Autodesk Fusion 360 part; units mm, degrees
(part 16 of 25)
  arc A4441 (68.687, 0.8538) -> (68.3831, 0.9459) centre (68.535, 0.8998) ccw
  line L1561 (83.8624, 50.0146) -> (84.0359, 50.3392)
  arc A4442 (68.3648, 3.5705) -> (68.6582, 3.692) centre (68.5115, 3.6312) ccw
  line L1562 (68.4422, 3.7777) -> (68.3972, 3.8451)
  arc A4443 (68.6582, 0.7615) -> (68.3648, 0.883) centre (68.5115, 0.8222) ccw
  arc A4444 (83.2647, 49.041) -> (83.0633, 49.2864) centre (83.164, 49.1637) ccw
  arc A4445 (33.749, 4.337) -> (33.749, 4.0195) centre (33.749, 4.1783) ccw
  line L1563 (67.8546, 4.1703) -> (67.7739, 4.1783)
  arc A4446 (33.3467, 3.8529) -> (33.1222, 4.0774) centre (33.2345, 3.9652) ccw
  line L1564 (33.1257, 3.8451) -> (33.0806, 3.7777)
  arc A4447 (67.839, 4.0124) -> (67.8702, 4.3283) centre (67.8546, 4.1704) ccw
  arc A4448 (32.8647, 3.692) -> (33.158, 3.5705) centre (33.0114, 3.6312) ccw
  line L1565 (33.0424, 3.7062) -> (33.0113, 3.6312)
  line L1566 (33.749, 4.1783) -> (33.6683, 4.1703)
  arc A4449 (32.9024, 3.781) -> (33.1824, 3.6313) centre (33.0424, 3.7062) ccw
  arc A4450 (32.8359, 3.5997) -> (33.1397, 3.5075) centre (32.9878, 3.5536) ccw
  line L1567 (68.0118, 4.131) -> (67.9342, 4.1545)
  arc A4451 (33.6527, 4.3283) -> (33.6838, 4.0124) centre (33.6683, 4.1704) ccw
  line L1568 (68.2257, 4.0166) -> (68.1582, 4.0617)
  arc A4452 (67.7894, 4.3363) -> (67.7583, 4.0203) centre (67.7739, 4.1783) ccw
  line L1569 (68.1582, 4.0617) -> (68.0867, 4.0999)
  arc A4453 (67.9802, 4.3064) -> (67.8881, 4.0026) centre (67.9341, 4.1545) ccw
  line L1570 (33.4362, 4.0999) -> (33.3646, 4.0617)
  line L1571 (33.0806, 3.7777) -> (33.0424, 3.7062)
  arc A4454 (33.2577, 3.7569) -> (32.9937, 3.9333) centre (33.1257, 3.8451) ccw
  arc A4455 (33.3754, 4.2466) -> (33.4969, 3.9533) centre (33.4361, 4.0999) ccw
  line L1572 (33.3646, 4.0617) -> (33.2972, 4.0166)
  arc A4456 (32.9486, 3.8659) -> (33.2126, 3.6895) centre (33.0806, 3.7777) ccw
  arc A4457 (68.2335, 3.7956) -> (68.458, 4.0201) centre (68.3458, 3.9079) ccw
  arc A4458 (33.3979, 3.8939) -> (33.1965, 4.1394) centre (33.2972, 4.0167) ccw
  arc A4459 (83.3016, 49.5247) -> (83.547, 49.3233) centre (83.4243, 49.424) ccw
  line L1573 (33.1771, 3.9078) -> (33.1257, 3.8451)
  arc A4460 (33.2998, 3.8071) -> (33.0544, 4.0085) centre (33.1771, 3.9078) ccw
  arc A4461 (33.6348, 4.0026) -> (33.5426, 4.3064) centre (33.5887, 4.1545) ccw
  arc A4462 (33.2206, 3.7029) -> (32.9406, 3.8525) centre (33.0806, 3.7777) ccw
  line L1574 (67.9342, 4.1545) -> (67.8546, 4.1703)
  arc A4463 (33.7645, 4.0203) -> (33.7334, 4.3363) centre (33.749, 4.1783) ccw
  arc A4464 (68.1375, 3.8846) -> (68.3139, 4.1486) centre (68.2257, 4.0166) ccw
  arc A4465 (67.7739, 4.0195) -> (67.7739, 4.337) centre (67.7739, 4.1783) ccw
  arc A4466 (68.0834, 3.9217) -> (68.2331, 4.2017) centre (68.1583, 4.0617) ccw
  arc A4467 (33.5718, 3.9843) -> (33.4503, 4.2776) centre (33.5111, 4.131) ccw
  arc A4468 (33.189, 3.6454) -> (32.8957, 3.7669) centre (33.0423, 3.7062) ccw
  arc A4469 (33.2898, 4.2017) -> (33.4395, 3.9217) centre (33.3646, 4.0617) ccw
  arc A4470 (33.511, 3.9599) -> (33.3613, 4.2399) centre (33.4362, 4.0999) ccw
  arc A4471 (33.6992, 4.0146) -> (33.6373, 4.326) centre (33.6683, 4.1703) ccw
  line L1575 (33.5887, 4.1545) -> (33.5111, 4.131)
  arc A4472 (33.209, 4.1486) -> (33.3854, 3.8846) centre (33.2972, 4.0166) ccw
  arc A4473 (68.0725, 4.2776) -> (67.951, 3.9843) centre (68.0118, 4.1309) ccw
  line L1576 (84.1767, 50.6793) -> (84.2253, 50.8394)
  arc A4474 (33.1633, 3.5852) -> (32.8594, 3.6773) centre (33.0114, 3.6312) ccw
  line L1577 (68.2884, 3.9652) -> (68.2257, 4.0166)
  arc A4475 (68.1615, 4.2399) -> (68.0119, 3.9599) centre (68.0867, 4.0999) ccw
  line L1578 (67.7739, 4.1783) -> (33.749, 4.1783)
  arc A4476 (67.9657, 3.9791) -> (68.0579, 4.2829) centre (68.0118, 4.131) ccw
  line L1579 (33.0113, 3.6312) -> (32.9878, 3.5536)
  arc A4477 (67.9032, 3.9988) -> (67.9651, 4.3102) centre (67.9342, 4.1545) ccw
  arc A4478 (33.465, 4.2829) -> (33.5572, 3.9791) centre (33.5111, 4.131) ccw
  arc A4479 (33.1338, 4.0879) -> (33.3352, 3.8425) centre (33.2345, 3.9652) ccw
  arc A4480 (33.4528, 3.9297) -> (33.2764, 4.1937) centre (33.3646, 4.0617) ccw
  arc A4481 (68.1877, 3.8425) -> (68.3891, 4.0879) centre (68.2884, 3.9652) ccw
  line L1580 (33.6683, 4.1703) -> (33.5887, 4.1545)
  line L1581 (33.2972, 4.0166) -> (33.2345, 3.9652)
  arc A4482 (68.3264, 4.1394) -> (68.125, 3.8939) centre (68.2257, 4.0166) ccw
  arc A4483 (33.0649, 4.0201) -> (33.2894, 3.7956) centre (33.1772, 3.9079) ccw
  line L1582 (33.2345, 3.9652) -> (33.1771, 3.9078)
  arc A4484 (68.026, 3.9533) -> (68.1475, 4.2466) centre (68.0867, 4.1) ccw
  arc A4485 (33.5577, 4.3102) -> (33.6197, 3.9988) centre (33.5887, 4.1545) ccw
  arc A4486 (1.1732, 49.6203) -> (1.4371, 49.7967) centre (1.3051, 49.7085) ccw
  line L1583 (0.7863, 50.6793) -> (0.9271, 50.3392)
  arc A4487 (0.9266, 50.7635) -> (0.6228, 50.6713) centre (0.7747, 50.7174) ccw
  arc A4488 (33.122, 1.0757) -> (32.806, 1.0446) centre (32.964, 1.0601) ccw
  line L1584 (32.964, 1.0601) -> (32.972, 0.9794)
  arc A4489 (0.9329, 50.7401) -> (0.6396, 50.6186) centre (0.7863, 50.6793) ccw
  arc A4490 (32.814, 0.9638) -> (33.13, 0.995) centre (32.972, 0.9794) ccw
  arc A4491 (32.806, 3.4089) -> (33.122, 3.3778) centre (32.964, 3.3933) ccw
  line L1585 (3.0543, 48.4113) -> (3.4066, 48.3044)
  line L1586 (1.1006, 50.0146) -> (1.3052, 49.7085)
  arc A4492 (1.6867, 49.0514) -> (1.9112, 49.2759) centre (1.799, 49.1637) ccw
  arc A4493 (32.8844, 0.7139) -> (33.1777, 0.8355) centre (33.0311, 0.7747) ccw
  arc A4494 (3.3605, 48.1525) -> (3.4527, 48.4563) centre (3.4066, 48.3044) ccw
  arc A4495 (33.13, 3.4585) -> (32.814, 3.4896) centre (32.972, 3.4741) ccw
  line L1587 (2.0835, 48.9302) -> (2.3896, 48.7256)
  line L1588 (1.5387, 49.424) -> (1.799, 49.1637)
  arc A4496 (1.8997, 49.2864) -> (1.6983, 49.041) centre (1.799, 49.1637) ccw
  arc A4497 (3.4375, 48.4601) -> (3.3756, 48.1487) centre (3.4065, 48.3044) ccw
  line L1589 (0.7747, 0.7747) -> (0.7747, 50.7174)
  arc A4498 (32.8321, 0.8689) -> (33.1435, 0.9308) centre (32.9878, 0.8998) ccw
  arc A4499 (33.031, 0.6159) -> (33.031, 0.9334) centre (33.031, 0.7747) ccw
  arc A4500 (1.2326, 50.1028) -> (0.9686, 49.9264) centre (1.1006, 50.0146) ccw
  arc A4501 (32.8594, 0.7761) -> (33.1633, 0.8683) centre (33.0114, 0.8222) ccw
  arc A4502 (68.2464, 4.1937) -> (68.07, 3.9297) centre (68.1582, 4.0617) ccw
  arc A4503 (33.003, 3.9458) -> (33.2484, 3.7444) centre (33.1257, 3.8451) ccw
  arc A4504 (33.158, 0.883) -> (32.8647, 0.7615) centre (33.0114, 0.8222) ccw
  arc A4505 (33.1397, 0.9459) -> (32.8359, 0.8538) centre (32.9878, 0.8999) ccw
  line L1590 (3.4066, 48.3044) -> (3.7676, 48.2326)
  arc A4506 (1.416, 49.3233) -> (1.6614, 49.5247) centre (1.5387, 49.424) ccw
  arc A4507 (1.9828, 48.8074) -> (2.1842, 49.0529) centre (2.0835, 48.9301) ccw
  arc A4508 (0.7805, 50.2785) -> (1.0738, 50.4) centre (0.9272, 50.3392) ccw
  line L1591 (2.3896, 48.7256) -> (2.7142, 48.5521)
  line L1592 (32.9878, 0.8998) -> (33.0113, 0.8222)
  arc A4509 (1.6509, 49.5362) -> (1.4264, 49.3117) centre (1.5387, 49.424) ccw
  arc A4510 (2.6394, 48.4121) -> (2.7891, 48.6921) centre (2.7143, 48.5521) ccw
  line L1593 (33.5111, 4.131) -> (33.4362, 4.0999)
  arc A4511 (3.7366, 48.0769) -> (3.7986, 48.3883) centre (3.7676, 48.2326) ccw
  arc A4512 (2.4644, 48.8656) -> (2.3148, 48.5856) centre (2.3896, 48.7256) ccw
  arc A4513 (33.1435, 3.5227) -> (32.8321, 3.5846) centre (32.9878, 3.5537) ccw
  line L1594 (1.799, 49.1637) -> (2.0835, 48.9302)
  arc A4514 (33.1277, 1.0104) -> (32.8163, 0.9484) centre (32.972, 0.9794) ccw
  line L1595 (2.7142, 48.5521) -> (3.0543, 48.4113)
  line L1596 (68.0867, 4.0999) -> (68.0118, 4.131)
  arc A4515 (1.4279, 49.8092) -> (1.1824, 49.6078) centre (1.3051, 49.7085) ccw
  arc A4516 (2.1717, 49.0621) -> (1.9953, 48.7982) centre (2.0835, 48.9302) ccw
  line L1597 (33.0113, 0.8222) -> (33.031, 0.7747)
  arc A4517 (32.8163, 3.505) -> (33.1277, 3.4431) centre (32.972, 3.474) ccw
  arc A4518 (32.8053, 1.0601) -> (33.1228, 1.0601) centre (32.9641, 1.0601) ccw
  line L1598 (33.031, 0.7747) -> (0.7747, 0.7747)
  arc A4519 (3.1004, 48.5632) -> (3.0082, 48.2593) centre (3.0543, 48.4113) ccw
  arc A4520 (2.3014, 48.5936) -> (2.4778, 48.8576) centre (2.3896, 48.7256) ccw
  arc A4521 (0.9334, 50.7174) -> (0.6159, 50.7174) centre (0.7747, 50.7174) ccw
  arc A4522 (67.8856, 4.326) -> (67.8236, 4.0146) centre (67.8546, 4.1703) ccw
  line L1599 (0.9271, 50.3392) -> (1.1006, 50.0146)
  arc A4523 (0.6343, 50.6332) -> (0.9382, 50.7254) centre (0.7863, 50.6793) ccw
  line L1600 (1.3052, 49.7085) -> (1.5387, 49.424)
  arc A4524 (2.9936, 48.2646) -> (3.1151, 48.5579) centre (3.0543, 48.4112) ccw
  arc A4525 (0.9606, 49.9398) -> (1.2406, 50.0894) centre (1.1006, 50.0146) ccw
  line L1601 (3.7676, 48.2326) -> (4.0005, 48.2096)
  arc A4526 (0.6159, 0.7747) -> (0.9334, 0.7747) centre (0.7747, 0.7747) ccw
  arc A4527 (33.1228, 3.3934) -> (32.8053, 3.3934) centre (32.9641, 3.3934) ccw
  arc A4528 (8.1085, 50.9855) -> (7.8047, 51.0777) centre (7.9566, 51.0316) ccw
  arc A4529 (8.0514, 52.1017) -> (8.0514, 52.4192) centre (8.0514, 52.2604) ccw
  arc A4530 (4.6199, 48.3676) -> (4.6511, 48.0517) centre (4.6355, 48.2097) ccw
  arc A4531 (3.9849, 48.0517) -> (4.0161, 48.3676) centre (4.0005, 48.2097) ccw
  arc A4532 (4.4768, 51.6255) -> (4.7943, 51.6255) centre (4.6356, 51.6255) ccw
  line L1602 (0.7747, 50.7174) -> (0.7863, 50.6793)
  arc A4533 (7.2096, 49.3117) -> (6.9851, 49.5362) centre (7.0974, 49.424) ccw
  arc A4534 (4.1593, 51.6255) -> (3.8418, 51.6255) centre (4.0005, 51.6255) ccw
  arc A4535 (4.4767, 48.2096) -> (4.7942, 48.2096) centre (4.6355, 48.2096) ccw
  arc A4536 (5.6278, 48.2593) -> (5.5356, 48.5632) centre (5.5817, 48.4113) ccw
  line L1603 (4.6355, 48.2096) -> (4.8684, 48.2326)
  line L1604 (4.0005, 48.2096) -> (4.0005, 51.6255)
  arc A4537 (1.0671, 50.4141) -> (0.7871, 50.2644) centre (0.9271, 50.3392) ccw
  arc A4538 (4.8839, 48.0746) -> (4.8528, 48.3906) centre (4.8683, 48.2326) ccw
  arc A4539 (7.3953, 50.0894) -> (7.6754, 49.9398) centre (7.5353, 50.0146) ccw
  arc A4540 (4.6355, 51.7843) -> (4.6355, 51.4668) centre (4.6355, 51.6256) ccw
  line L1605 (4.6355, 51.6255) -> (4.6355, 52.2605)
  line L1606 (7.9566, 51.0316) -> (8.0284, 51.3926)
  arc A4541 (7.9964, 50.6186) -> (7.7031, 50.7401) centre (7.8498, 50.6793) ccw
  arc A4542 (4.0005, 51.7842) -> (4.0005, 51.4667) centre (4.0005, 51.6255) ccw
  arc A4543 (3.7832, 48.3906) -> (3.752, 48.0746) centre (3.7676, 48.2326) ccw
  line L1607 (5.5817, 48.4113) -> (5.9218, 48.5521)
  arc A4544 (4.7943, 52.2605) -> (4.4768, 52.2605) centre (4.6356, 52.2605) ccw
  line L1608 (4.6355, 52.2605) -> (8.0514, 52.2605)
  arc A4545 (4.6355, 51.4667) -> (4.6355, 51.7842) centre (4.6355, 51.6255) ccw
  line L1609 (4.0005, 51.6255) -> (4.6355, 51.6255)
  line L1610 (32.972, 0.9794) -> (32.9878, 0.8998)
  arc A4546 (6.3212, 48.5856) -> (6.1716, 48.8656) centre (6.2464, 48.7256) ccw
  line L1611 (6.2464, 48.7256) -> (6.5525, 48.9302)
  arc A4547 (6.9746, 49.5247) -> (7.22, 49.3233) centre (7.0973, 49.424) ccw
  arc A4548 (5.8469, 48.6921) -> (5.9966, 48.4121) centre (5.9218, 48.5521) ccw
  arc A4549 (8.2093, 51.6099) -> (7.8934, 51.6411) centre (8.0513, 51.6255) ccw
  arc A4550 (6.4518, 49.0529) -> (6.6532, 48.8074) centre (6.5525, 48.9301) ccw
  line L1612 (32.964, 3.3934) -> (32.964, 1.0601)
  arc A4551 (7.8704, 51.4082) -> (8.1864, 51.377) centre (8.0284, 51.3926) ccw
  arc A4552 (3.8418, 48.2096) -> (4.1593, 48.2096) centre (4.0005, 48.2096) ccw
  line L1613 (7.8497, 50.6793) -> (7.9566, 51.0316)
  line L1614 (7.3308, 49.7085) -> (7.5354, 50.0146)
  arc A4553 (5.5209, 48.5579) -> (5.6424, 48.2646) centre (5.5816, 48.4112) ccw
  arc A4554 (8.1841, 51.3616) -> (7.8727, 51.4236) centre (8.0284, 51.3926) ccw
  arc A4555 (4.8374, 48.3883) -> (4.8994, 48.0769) centre (4.8684, 48.2326) ccw
  arc A4556 (7.8009, 51.0625) -> (8.1123, 51.0006) centre (7.9566, 51.0316) ccw
  line L1615 (5.2294, 48.3044) -> (5.5817, 48.4113)
  arc A4557 (7.8489, 50.2644) -> (7.5689, 50.4141) centre (7.7089, 50.3392) ccw
  arc A4558 (0.7747, 0.9334) -> (0.7747, 0.6159) centre (0.7747, 0.7747) ccw
  arc A4559 (7.6978, 50.7254) -> (8.0017, 50.6332) centre (7.8498, 50.6793) ccw
  line L1616 (32.9878, 3.5536) -> (32.972, 3.4741)
  line L1617 (7.5354, 50.0146) -> (7.7089, 50.3392)
  arc A4560 (8.0514, 51.4668) -> (8.0514, 51.7843) centre (8.0514, 51.6256) ccw
  line L1618 (32.972, 3.4741) -> (32.964, 3.3934)
  line L1619 (5.9218, 48.5521) -> (6.2464, 48.7256)
  line L1620 (8.0284, 51.3926) -> (8.0514, 51.6255)
  line L1621 (8.0514, 51.6255) -> (4.6355, 51.6255)
  arc A4561 (6.7248, 49.2759) -> (6.9493, 49.0514) centre (6.8371, 49.1637) ccw
  line L1622 (4.8684, 48.2326) -> (5.2294, 48.3044)
  arc A4562 (5.1833, 48.4563) -> (5.2755, 48.1525) centre (5.2294, 48.3044) ccw
  arc A4563 (2.775, 48.6988) -> (2.6535, 48.4055) centre (2.7143, 48.5522) ccw
  arc A4564 (5.2604, 48.1487) -> (5.1985, 48.4601) centre (5.2294, 48.3044) ccw
  line L1623 (6.837, 49.1637) -> (7.0973, 49.424)
  arc A4565 (4.7942, 51.6255) -> (4.4767, 51.6255) centre (4.6355, 51.6255) ccw
  line L1624 (7.0973, 49.424) -> (7.3308, 49.7085)
  arc A4566 (7.6673, 49.9264) -> (7.4034, 50.1028) centre (7.5353, 50.0146) ccw
  arc A4567 (71.3694, 40.4649) -> (71.3694, 40.7824) centre (71.3694, 40.6237) ccw
  line L1625 (70.4098, 40.4328) -> (70.3249, 40.3479)
  arc A4568 (7.4536, 49.6078) -> (7.2081, 49.8092) centre (7.3309, 49.7085) ccw
  arc A4569 (5.4611, 55.6772) -> (5.3689, 55.3734) centre (5.415, 55.5253) ccw
  arc A4570 (6.4643, 54.8238) -> (6.6407, 55.0878) centre (6.5525, 54.9558) ccw
  arc A4571 (72.227, 39.5586) -> (72.5204, 39.6801) centre (72.3737, 39.6194) ccw
  arc A4572 (70.3491, 40.5795) -> (70.4706, 40.2862) centre (70.4099, 40.4329) ccw
  arc A4573 (7.6754, 53.9462) -> (7.3953, 53.7966) centre (7.5353, 53.8714) ccw
  arc A4574 (6.6532, 55.0786) -> (6.4518, 54.8331) centre (6.5525, 54.9558) ccw
  line L1626 (6.837, 54.7223) -> (6.5525, 54.9558)
  line L1627 (7.7089, 53.5468) -> (7.5354, 53.8714)
  line L1628 (4.6355, 51.6255) -> (4.6355, 48.2096)
  arc A4575 (6.3346, 55.2923) -> (6.1582, 55.0284) centre (6.2464, 55.1604) ccw
  line L1629 (6.2464, 55.1604) -> (5.9218, 55.3339)
  arc A4576 (7.8555, 53.6075) -> (7.5622, 53.486) centre (7.7088, 53.5468) ccw
  arc A4577 (7.22, 54.5627) -> (6.9746, 54.3613) centre (7.0973, 54.462) ccw
  line L1630 (5.9218, 55.3339) -> (5.5817, 55.4747)
  arc A4578 (5.6424, 55.6214) -> (5.5209, 55.3281) centre (5.5816, 55.4748) ccw
  arc A4579 (6.6407, 48.7982) -> (6.4643, 49.0621) centre (6.5525, 48.9301) ccw
  arc A4580 (7.4628, 54.2657) -> (7.1988, 54.0893) centre (7.3308, 54.1775) ccw
  arc A4581 (70.8706, 40.7824) -> (70.8706, 40.4649) centre (70.8706, 40.6237) ccw
  arc A4582 (70.2126, 40.4602) -> (70.4372, 40.2356) centre (70.3249, 40.3479) ccw
  arc A4583 (8.0017, 53.2528) -> (7.6978, 53.1606) centre (7.8497, 53.2067) ccw
  line L1631 (6.5525, 54.9558) -> (6.2464, 55.1604)
  line L1632 (7.5354, 53.8714) -> (7.3308, 54.1775)
  arc A4584 (7.8934, 52.2449) -> (8.2093, 52.2761) centre (8.0514, 52.2605) ccw
  arc A4585 (6.1582, 48.8576) -> (6.3346, 48.5936) centre (6.2464, 48.7256) ccw
  arc A4586 (72.0706, 39.9679) -> (72.2951, 40.1924) centre (72.1829, 40.0802) ccw
  arc A4587 (8.1123, 52.8854) -> (7.8009, 52.8235) centre (7.9566, 52.8545) ccw
  line L1633 (70.8706, 40.6237) -> (70.4098, 40.4328)
  arc A4588 (6.7363, 54.5996) -> (6.9377, 54.845) centre (6.837, 54.7223) ccw
  line L1634 (8.0284, 52.4934) -> (7.9566, 52.8544)
  arc A4589 (6.9377, 49.041) -> (6.7363, 49.2864) centre (6.837, 49.1637) ccw
  arc A4590 (70.5221, 40.3206) -> (70.2976, 40.5451) centre (70.4099, 40.4329) ccw
  arc A4591 (8.1864, 52.5089) -> (7.8704, 52.4778) centre (8.0284, 52.4934) ccw
  arc A4592 (7.5689, 53.4719) -> (7.8489, 53.6216) centre (7.7089, 53.5468) ccw
  arc A4593 (7.7031, 53.1459) -> (7.9964, 53.2674) centre (7.8498, 53.2067) ccw
  line L1635 (5.5817, 55.4747) -> (5.415, 55.5253)
  arc A4594 (6.9493, 54.8346) -> (6.7248, 54.6101) centre (6.8371, 54.7224) ccw
  arc A4595 (72.2149, 39.1206) -> (72.5324, 39.1206) centre (72.3736, 39.1206) ccw
  arc A4596 (5.9825, 48.4055) -> (5.861, 48.6988) centre (5.9218, 48.5522) ccw
  arc A4597 (7.8727, 52.4624) -> (8.1841, 52.5244) centre (8.0284, 52.4934) ccw
  arc A4598 (5.9966, 55.4739) -> (5.8469, 55.1939) centre (5.9217, 55.3339) ccw
  line L1636 (8.0514, 52.2605) -> (8.0284, 52.4934)
  arc A4599 (5.861, 55.1872) -> (5.9825, 55.4805) centre (5.9218, 55.3338) ccw
  arc A4600 (70.9314, 40.477) -> (70.8099, 40.7704) centre (70.8706, 40.6237) ccw
  line L1637 (5.415, 55.5253) -> (79.548, 55.5253)
  arc A4601 (5.5356, 55.3228) -> (5.6278, 55.6267) centre (5.5817, 55.4748) ccw
  arc A4602 (7.5622, 50.4) -> (7.8555, 50.2785) centre (7.7088, 50.3392) ccw
  line L1638 (71.3694, 40.6237) -> (70.8706, 40.6237)
  line L1639 (7.7089, 50.3392) -> (7.8497, 50.6793)
  line L1640 (7.3308, 54.1775) -> (7.0973, 54.462)
  line L1641 (72.3737, 39.1206) -> (72.3737, 39.6194)
  arc A4603 (72.5324, 39.6194) -> (72.2149, 39.6194) centre (72.3736, 39.6194) ccw
  line L1642 (6.5525, 48.9302) -> (6.837, 49.1637)
  arc A4604 (4.6355, 52.4192) -> (4.6355, 52.1017) centre (4.6355, 52.2604) ccw
  line L1643 (7.0973, 54.462) -> (6.837, 54.7223)
  arc A4605 (79.548, 55.3666) -> (79.548, 55.684) centre (79.548, 55.5253) ccw
  arc A4606 (7.1988, 49.7967) -> (7.4628, 49.6203) centre (7.3308, 49.7085) ccw
  line L1644 (72.3737, 39.6194) -> (72.1828, 40.0802)
  arc A4607 (7.8047, 52.8083) -> (8.1085, 52.9005) centre (7.9566, 52.8544) ccw
  arc A4608 (72.3295, 40.1409) -> (72.0362, 40.0194) centre (72.1829, 40.0802) ccw
  line L1645 (52.2859, 37.4845) -> (52.2859, 38.2029)
  arc A4609 (52.4446, 38.2029) -> (52.1271, 38.2029) centre (52.2858, 38.2029) ccw
  line L1646 (52.2859, 38.2029) -> (52.4751, 38.3921)
  arc A4610 (51.9362, 40.2012) -> (51.8147, 40.4946) centre (51.8755, 40.3479) ccw
  arc A4611 (50.0723, 36.5018) -> (50.2968, 36.7264) centre (50.1845, 36.6141) ccw
  arc A4612 (6.1716, 55.0203) -> (6.3212, 55.3004) centre (6.2464, 55.1604) ccw
  arc A4613 (71.7694, 40.2862) -> (71.8909, 40.5795) centre (71.8302, 40.4329) ccw
  arc A4614 (52.1271, 37.4845) -> (52.4446, 37.4845) centre (52.2858, 37.4845) ccw
  line L1647 (50.9029, 39.5859) -> (50.1845, 39.5859)
  line L1648 (52.4751, 38.3921) -> (70.3249, 38.3921)
  arc A4615 (70.3249, 38.2334) -> (70.3249, 38.5508) centre (70.3249, 38.3921) ccw
  arc A4616 (52.4751, 38.5508) -> (52.4751, 38.2334) centre (52.4751, 38.3921) ccw
  line L1649 (72.1828, 38.6598) -> (72.3737, 39.1206)
  line L1650 (71.3694, 38.1163) -> (71.8302, 38.3072)
  arc A4617 (50.1845, 36.7728) -> (50.1845, 36.4554) centre (50.1845, 36.6141) ccw
  arc A4618 (52.5873, 38.2798) -> (52.3628, 38.5044) centre (52.4751, 38.3921) ccw
  arc A4619 (52.3982, 37.3723) -> (52.1736, 37.5968) centre (52.2859, 37.4846) ccw
  arc A4620 (51.6283, 40.0868) -> (51.4038, 40.3113) centre (51.516, 40.199) ccw
  arc A4621 (52.1736, 38.3152) -> (52.3982, 38.0907) centre (52.2859, 38.203) ccw
  arc A4622 (70.4372, 38.5044) -> (70.2126, 38.2798) centre (70.3249, 38.3921) ccw
  arc A4623 (51.4155, 36.4554) -> (51.4155, 36.7728) centre (51.4155, 36.6141) ccw
  arc A4624 (49.4264, 37.5968) -> (49.2018, 37.3723) centre (49.3141, 37.4846) ccw
  line L1651 (70.4098, 38.3072) -> (70.8706, 38.1163)
  line L1652 (50.1845, 36.6141) -> (51.4155, 36.6141)
  arc A4625 (70.4706, 38.4538) -> (70.3491, 38.1605) centre (70.4099, 38.3072) ccw
  arc A4626 (70.8099, 37.9696) -> (70.9314, 38.263) centre (70.8706, 38.1163) ccw
  arc A4627 (50.7907, 39.6982) -> (51.0152, 39.4736) centre (50.903, 39.5859) ccw
  line L1653 (53.34, 17.78) -> (53.34, 19.2405)
  line L1654 (53.34, 19.2405) -> (53.34, 17.78)
  line L1655 (71.8302, 40.4328) -> (71.3694, 40.6237)
  line L1656 (51.5161, 40.199) -> (51.241, 39.9239)
  arc A4628 (71.4301, 40.7704) -> (71.3086, 40.477) centre (71.3693, 40.6237) ccw
  line L1657 (7.9566, 52.8544) -> (7.8497, 53.2067)
  arc A4629 (70.8706, 38.2751) -> (70.8706, 37.9576) centre (70.8706, 38.1164) ccw
  arc A4630 (72.2951, 38.5476) -> (72.0706, 38.7721) centre (72.1829, 38.6599) ccw
  line L1658 (51.8755, 40.3479) -> (51.5161, 40.199)
  line L1659 (70.8706, 38.1163) -> (71.3694, 38.1163)
  line L1660 (7.8497, 53.2067) -> (7.7089, 53.5468)
  arc A4631 (71.7179, 38.4194) -> (71.9424, 38.1949) centre (71.8302, 38.3072) ccw
  arc A4632 (49.2018, 38.8277) -> (49.4264, 38.6032) centre (49.3141, 38.7155) ccw
  arc A4633 (53.4988, 19.2405) -> (53.1813, 19.2405) centre (53.3401, 19.2405) ccw
  arc A4634 (70.3249, 40.1891) -> (70.3249, 40.5066) centre (70.3249, 40.3479) ccw
  arc A4635 (51.1287, 40.0362) -> (51.3532, 39.8117) centre (51.241, 39.924) ccw
  arc A4636 (71.3086, 38.263) -> (71.4301, 37.9696) centre (71.3693, 38.1163) ccw
  arc A4637 (50.9029, 39.4271) -> (50.9029, 39.7446) centre (50.9029, 39.5859) ccw
  arc A4638 (7.4034, 53.7832) -> (7.6673, 53.9596) centre (7.5353, 53.8714) ccw
  arc A4639 (51.3532, 39.8117) -> (51.1287, 40.0362) centre (51.241, 39.924) ccw
  arc A4640 (70.2976, 38.1949) -> (70.5221, 38.4194) centre (70.4099, 38.3072) ccw
  arc A4641 (7.2081, 54.0768) -> (7.4536, 54.2782) centre (7.3308, 54.1775) ccw
  arc A4642 (71.9424, 40.5451) -> (71.7179, 40.3206) centre (71.8302, 40.4328) ccw
  line L1661 (72.1828, 40.0802) -> (71.8302, 40.4328)
  arc A4643 (5.415, 55.684) -> (5.415, 55.3666) centre (5.415, 55.5253) ccw
  arc A4644 (51.8755, 40.5066) -> (51.8755, 40.1891) centre (51.8755, 40.3479) ccw
  arc A4645 (71.3694, 37.9576) -> (71.3694, 38.2751) centre (71.3694, 38.1164) ccw
  arc A4646 (6.9851, 54.3498) -> (7.2096, 54.5743) centre (7.0974, 54.4621) ccw
  line L1662 (49.3141, 37.4845) -> (50.1845, 36.6141)
  arc A4647 (50.2968, 39.4736) -> (50.0723, 39.6982) centre (50.1846, 39.5859) ccw
  arc A4648 (50.1845, 39.7446) -> (50.1845, 39.4271) centre (50.1845, 39.5859) ccw
  arc A4649 (51.3032, 36.7264) -> (51.5277, 36.5018) centre (51.4154, 36.6141) ccw
  arc A4650 (53.4987, 19.2405) -> (53.1812, 19.2405) centre (53.34, 19.2405) ccw
  line L1663 (70.3249, 40.3479) -> (51.8755, 40.3479)
  line L1664 (51.241, 39.9239) -> (50.9029, 39.5859)
  line L1665 (50.1845, 39.5859) -> (49.3141, 38.7155)
  arc A4651 (28.1833, 34.8511) -> (28.4079, 35.0756) centre (28.2956, 34.9634) ccw
  arc A4652 (53.945, 19.0817) -> (53.945, 19.3992) centre (53.945, 19.2405) ccw
  arc A4653 (53.34, 17.9388) -> (53.34, 17.6213) centre (53.34, 17.78) ccw
  line L1666 (49.3141, 38.7155) -> (49.3141, 37.4845)
  arc A4654 (16.5671, 14.6245) -> (16.8846, 14.6245) centre (16.7259, 14.6245) ccw
  line L1667 (25.0444, 37.4267) -> (25.6921, 36.779)
  line L1668 (27.3433, 39.7256) -> (25.9967, 39.7256)
  line L1669 (25.0444, 34.9633) -> (25.0444, 33.6167)
  arc A4655 (51.7104, 19.0868) -> (51.8319, 19.3801) centre (51.7712, 19.2334) ccw
  arc A4656 (27.4891, 35.611) -> (27.8066, 35.611) centre (27.6479, 35.611) ccw
  arc A4657 (28.4543, 34.9633) -> (28.1368, 34.9633) centre (28.2956, 34.9633) ccw
  line L1670 (70.3249, 38.3921) -> (70.4098, 38.3072)
  arc A4658 (25.5798, 36.6667) -> (25.8044, 36.8912) centre (25.6921, 36.779) ccw
  line L1671 (52.2496, 18.7551) -> (51.7712, 19.2335)
  line L1672 (50.459, 19.4945) -> (49.8288, 19.2335)
  line L1673 (52.735, 19.2405) -> (52.2496, 18.7551)
  arc A4659 (46.4368, 21.5237) -> (46.6613, 21.7482) centre (46.549, 21.636) ccw
  arc A4660 (27.3433, 39.5668) -> (27.3433, 39.8843) centre (27.3433, 39.7256) ccw
  arc A4661 (72.0362, 38.7206) -> (72.3295, 38.5991) centre (72.1829, 38.6599) ccw
  arc A4662 (46.2739, 22.0698) -> (46.2739, 21.7523) centre (46.2739, 21.9111) ccw
  arc A4663 (25.5333, 35.611) -> (25.8509, 35.611) centre (25.6921, 35.611) ccw
  line L1674 (25.6921, 36.779) -> (25.6921, 35.611)
  line L1675 (28.2956, 38.7733) -> (27.3433, 39.7256)
  arc A4664 (25.8044, 35.4988) -> (25.5798, 35.7233) centre (25.6921, 35.6111) ccw
  arc A4665 (28.1368, 37.4267) -> (28.4543, 37.4267) centre (28.2956, 37.4267) ccw
  arc A4666 (24.8856, 33.6167) -> (25.2032, 33.6167) centre (25.0444, 33.6167) ccw
  arc A4667 (72.5204, 39.0599) -> (72.227, 39.1814) centre (72.3737, 39.1206) ccw
  arc A4668 (50.459, 19.6532) -> (50.459, 19.3357) centre (50.459, 19.4945) ccw
  arc A4669 (51.141, 19.3357) -> (51.141, 19.6532) centre (51.141, 19.4945) ccw
  arc A4670 (51.8834, 19.3457) -> (51.6589, 19.1212) centre (51.7712, 19.2335) ccw
  line L1676 (27.3433, 32.6644) -> (28.2956, 33.6167)
  arc A4671 (27.2311, 32.7767) -> (27.4556, 32.5521) centre (27.3434, 32.6644) ccw
  arc A4672 (28.1368, 33.6167) -> (28.4543, 33.6167) centre (28.2956, 33.6167) ccw
  arc A4673 (52.1373, 18.6428) -> (52.3619, 18.8673) centre (52.2496, 18.755) ccw
  arc A4674 (49.7681, 19.3801) -> (49.8896, 19.0868) centre (49.8289, 19.2335) ccw
  arc A4675 (50.5197, 19.3478) -> (50.3982, 19.6412) centre (50.459, 19.4945) ccw
  line L1677 (51.7712, 19.2335) -> (51.141, 19.4945)
  arc A4676 (52.735, 19.3992) -> (52.735, 19.0817) centre (52.735, 19.2405) ccw
  arc A4677 (51.2018, 19.6412) -> (51.0803, 19.3478) centre (51.1411, 19.4945) ccw
  line L1678 (71.8302, 38.3072) -> (72.1828, 38.6598)
  arc A4678 (49.1554, 37.4845) -> (49.4729, 37.4845) centre (49.3142, 37.4845) ccw
  arc A4679 (27.8066, 36.779) -> (27.4891, 36.779) centre (27.6479, 36.779) ccw
  line L1679 (27.6479, 36.779) -> (28.2956, 37.4267)
  line L1680 (51.141, 19.4945) -> (50.459, 19.4945)
  arc A4680 (52.8473, 19.1282) -> (52.6228, 19.3528) centre (52.7351, 19.2405) ccw
  arc A4681 (53.1813, 17.78) -> (53.4988, 17.78) centre (53.3401, 17.78) ccw
  line L1681 (51.4155, 36.6141) -> (52.2859, 37.4845)
  arc A4682 (53.34, 19.0817) -> (53.34, 19.3992) centre (53.34, 19.2405) ccw
  arc A4683 (71.8909, 38.1605) -> (71.7694, 38.4538) centre (71.8302, 38.3072) ccw
  arc A4684 (52.1373, 18.8673) -> (52.3619, 18.6428) centre (52.2496, 18.7551) ccw
  line L1682 (53.34, 19.2405) -> (52.735, 19.2405)
  arc A4685 (53.1812, 17.78) -> (53.4987, 17.78) centre (53.34, 17.78) ccw
  arc A4686 (27.4556, 39.8379) -> (27.2311, 39.6133) centre (27.3434, 39.7256) ccw
  arc A4687 (12.7062, 34.7907) -> (12.4129, 34.9122) centre (12.5596, 34.8514) ccw
  arc A4688 (49.4729, 38.7155) -> (49.1554, 38.7155) centre (49.3142, 38.7155) ccw
  arc A4689 (14.6245, 16.8846) -> (14.6245, 16.5671) centre (14.6245, 16.7259) ccw
  arc A4690 (51.4553, 40.3457) -> (51.5768, 40.0524) centre (51.516, 40.1991) ccw
  arc A4691 (53.34, 17.6213) -> (53.34, 17.9388) centre (53.34, 17.78) ccw
  line L1683 (25.9967, 32.6644) -> (27.3433, 32.6644)
  line L1684 (15.8555, 16.7259) -> (14.6245, 16.7259)
  arc A4692 (14.7368, 16.6136) -> (14.5123, 16.8382) centre (14.6245, 16.7259) ccw
  arc A4693 (15.9677, 16.8382) -> (15.7432, 16.6136) centre (15.8555, 16.7259) ccw
  arc A4694 (16.8846, 15.8555) -> (16.5671, 15.8555) centre (16.7259, 15.8555) ccw
  line L1685 (7.62, 21.59) -> (7.62, 23.4315)
  line L1686 (14.6245, 16.7259) -> (13.7541, 15.8555)
  arc A4695 (7.7787, 21.59) -> (7.4612, 21.59) centre (7.62, 21.59) ccw
  line L1687 (13.7541, 15.8555) -> (13.7541, 14.6245)
  line L1688 (5.7785, 22.3528) -> (5.7785, 21.59)
  arc A4696 (13.6418, 15.9677) -> (13.8664, 15.7432) centre (13.7541, 15.8554) ccw
  arc A4697 (28.1833, 38.6611) -> (28.4079, 38.8856) centre (28.2956, 38.7734) ccw
  arc A4698 (15.8555, 13.5954) -> (15.8555, 13.9129) centre (15.8555, 13.7542) ccw
  arc A4699 (9.3027, 20.8272) -> (9.6202, 20.8272) centre (9.4615, 20.8272) ccw
  line L1689 (6.8572, 23.4315) -> (5.7785, 22.3528)
  line L1690 (25.9967, 39.7256) -> (25.0444, 38.7733)
  arc A4700 (25.9967, 39.8843) -> (25.9967, 39.5668) centre (25.9967, 39.7256) ccw
  line L1691 (25.0444, 38.7733) -> (25.0444, 37.4267)
  arc A4701 (25.1567, 33.7289) -> (24.9321, 33.5044) centre (25.0444, 33.6167) ccw
  arc A4702 (7.62, 21.4312) -> (7.62, 21.7487) centre (7.62, 21.59) ccw
  arc A4703 (25.8509, 36.779) -> (25.5333, 36.779) centre (25.6921, 36.779) ccw
  arc A4704 (25.8844, 32.5521) -> (26.1089, 32.7767) centre (25.9966, 32.6644) ccw
  arc A4705 (28.4079, 37.3144) -> (28.1833, 37.5389) centre (28.2956, 37.4267) ccw
  arc A4706 (24.9321, 38.8856) -> (25.1567, 38.6611) centre (25.0444, 38.7734) ccw
  arc A4707 (28.4543, 38.7733) -> (28.1368, 38.7733) centre (28.2956, 38.7733) ccw
  line L1692 (25.6921, 35.611) -> (25.0444, 34.9633)
  arc A4708 (26.1089, 39.6133) -> (25.8844, 39.8379) centre (25.9966, 39.7256) ccw
  arc A4709 (27.3433, 32.5057) -> (27.3433, 32.8231) centre (27.3433, 32.6644) ccw
  arc A4710 (25.2032, 34.9633) -> (24.8856, 34.9633) centre (25.0444, 34.9633) ccw
  line L1693 (27.6479, 35.611) -> (27.6479, 36.779)
  arc A4711 (16.6136, 15.7432) -> (16.8382, 15.9677) centre (16.7259, 15.8554) ccw
  arc A4712 (25.9967, 32.8231) -> (25.9967, 32.5057) centre (25.9967, 32.6644) ccw
  line L1694 (28.2956, 33.6167) -> (28.2956, 34.9633)
  line L1695 (16.7259, 14.6245) -> (16.7259, 15.8555)
  arc A4713 (27.7602, 35.7233) -> (27.5356, 35.4988) centre (27.6479, 35.611) ccw
  arc A4714 (24.9321, 35.0756) -> (25.1567, 34.8511) centre (25.0444, 34.9634) ccw
  line L1696 (16.7259, 15.8555) -> (15.8555, 16.7259)
  line L1697 (28.2956, 37.4267) -> (28.2956, 38.7733)
  arc A4715 (25.2032, 38.7733) -> (24.8856, 38.7733) centre (25.0444, 38.7733) ccw
  arc A4716 (24.8856, 37.4267) -> (25.2032, 37.4267) centre (25.0444, 37.4267) ccw
  arc A4717 (13.8664, 14.7368) -> (13.6418, 14.5123) centre (13.7541, 14.6246) ccw
  arc A4718 (7.4612, 19.7485) -> (7.7787, 19.7485) centre (7.62, 19.7485) ccw
  line L1698 (9.4615, 21.59) -> (9.4615, 22.3528)
  arc A4719 (5.6662, 22.465) -> (5.8908, 22.2405) centre (5.7785, 22.3528) ccw
  arc A4720 (25.1567, 37.5389) -> (24.9321, 37.3144) centre (25.0444, 37.4267) ccw
  arc A4721 (6.9695, 23.3192) -> (6.745, 23.5438) centre (6.8573, 23.4315) ccw
  arc A4722 (28.4079, 33.5044) -> (28.1833, 33.7289) centre (28.2956, 33.6167) ccw
  line L1699 (25.0444, 33.6167) -> (25.9967, 32.6644)
  line L1700 (14.6245, 13.7541) -> (15.8555, 13.7541)
  arc A4723 (7.4612, 21.59) -> (7.7787, 21.59) centre (7.62, 21.59) ccw
  line L1701 (7.62, 19.7485) -> (8.3828, 19.7485)
  arc A4724 (7.62, 21.7488) -> (7.62, 21.4313) centre (7.62, 21.5901) ccw
  arc A4725 (27.5356, 36.8912) -> (27.7602, 36.6667) centre (27.6479, 36.7789) ccw
  arc A4726 (7.7788, 23.4315) -> (7.4613, 23.4315) centre (7.6201, 23.4315) ccw
  arc A4727 (6.8572, 19.9073) -> (6.8572, 19.5897) centre (6.8572, 19.7485) ccw
  line L1702 (7.62, 21.59) -> (9.4615, 21.59)
  line L1703 (8.3828, 19.7485) -> (9.4615, 20.8272)
  line L1704 (28.2956, 34.9633) -> (27.6479, 35.611)
  arc A4728 (15.8555, 16.5671) -> (15.8555, 16.8846) centre (15.8555, 16.7259) ccw
  line L1705 (9.4615, 20.8272) -> (9.4615, 21.59)
  arc A4729 (8.495, 23.5438) -> (8.2705, 23.3192) centre (8.3827, 23.4315) ccw
  arc A4730 (14.5123, 13.6418) -> (14.7368, 13.8664) centre (14.6246, 13.7541) ccw
  arc A4731 (7.4613, 21.59) -> (7.7788, 21.59) centre (7.6201, 21.59) ccw
  arc A4732 (9.4615, 21.4312) -> (9.4615, 21.7487) centre (9.4615, 21.59) ccw
  arc A4733 (15.7432, 13.8664) -> (15.9677, 13.6418) centre (15.8554, 13.7541) ccw
  line L1706 (15.2918, 24.8452) -> (15.7526, 24.6543)
  arc A4734 (7.4613, 19.7485) -> (7.7788, 19.7485) centre (7.6201, 19.7485) ccw
  line L1707 (14.7483, 26.1574) -> (14.7483, 25.6586)
  line L1708 (13.7541, 14.6245) -> (14.6245, 13.7541)
  arc A4735 (7.62, 21.4313) -> (7.62, 21.7488) centre (7.62, 21.5901) ccw
  arc A4736 (8.2705, 19.8608) -> (8.495, 19.6362) centre (8.3827, 19.7485) ccw
  line L1709 (9.4615, 21.59) -> (7.62, 21.59)
  arc A4737 (7.62, 23.2727) -> (7.62, 23.5902) centre (7.62, 23.4315) ccw
  arc A4738 (7.62, 21.4312) -> (7.62, 21.7487) centre (7.62, 21.59) ccw
  arc A4739 (15.7526, 24.8131) -> (15.7526, 24.4956) centre (15.7526, 24.6543) ccw
  arc A4740 (5.7785, 21.7488) -> (5.7785, 21.4313) centre (5.7785, 21.5901) ccw
  arc A4741 (7.4613, 21.59) -> (7.7788, 21.59) centre (7.6201, 21.59) ccw
  arc A4742 (5.6197, 21.59) -> (5.9373, 21.59) centre (5.7785, 21.59) ccw
  line L1710 (8.6955, 26.9621) -> (15.2831, 26.9621)
  arc A4743 (13.9129, 15.8555) -> (13.5954, 15.8555) centre (13.7542, 15.8555) ccw
  arc A4744 (7.62, 21.7488) -> (7.62, 21.4313) centre (7.62, 21.5901) ccw
  arc A4745 (7.62, 21.7487) -> (7.62, 21.4312) centre (7.62, 21.59) ccw
  arc A4746 (7.7788, 21.59) -> (7.4613, 21.59) centre (7.6201, 21.59) ccw
  arc A4747 (9.3027, 21.59) -> (9.6202, 21.59) centre (9.4615, 21.59) ccw
  line L1711 (8.488, 31.3055) -> (6.752, 31.3055)
  arc A4748 (9.3492, 22.2405) -> (9.5738, 22.465) centre (9.4615, 22.3527) ccw
  arc A4749 (5.4122, 30.1902) -> (5.6368, 29.9657) centre (5.5245, 30.078) ccw
  arc A4750 (9.6032, 29.9657) -> (9.8278, 30.1902) centre (9.7155, 30.078) ccw
  arc A4751 (8.3828, 23.2727) -> (8.3828, 23.5902) centre (8.3828, 23.4315) ccw
  arc A4752 (7.62, 19.9073) -> (7.62, 19.5897) centre (7.62, 19.7485) ccw
  arc A4753 (9.5738, 20.715) -> (9.3492, 20.9395) centre (9.4615, 20.8272) ccw
  line L1712 (7.62, 19.7485) -> (7.62, 21.59)
  line L1713 (7.62, 23.4315) -> (6.8572, 23.4315)
  arc A4754 (8.4448, 27.2267) -> (8.2202, 27.0023) centre (8.3325, 27.1145) ccw
  arc A4755 (7.62, 21.7487) -> (7.62, 21.4312) centre (7.62, 21.59) ccw
  line L1714 (15.7526, 24.6543) -> (16.2514, 24.6543)
  arc A4756 (8.3968, 27.2576) -> (8.2753, 26.9643) centre (8.3361, 27.111) ccw
  line L1715 (8.3828, 23.4315) -> (7.62, 23.4315)
  arc A4757 (6.8572, 23.5902) -> (6.8572, 23.2727) centre (6.8572, 23.4315) ccw
  arc A4758 (8.3325, 26.9557) -> (8.3325, 27.2733) centre (8.3325, 27.1145) ccw
  line L1716 (7.62, 21.59) -> (7.62, 19.7485)
  arc A4759 (9.4615, 21.4313) -> (9.4615, 21.7488) centre (9.4615, 21.5901) ccw
  arc A4760 (7.62, 19.5897) -> (7.62, 19.9073) centre (7.62, 19.7485) ccw
  arc A4761 (9.6202, 22.3528) -> (9.3027, 22.3528) centre (9.4615, 22.3528) ccw
  arc A4762 (16.8382, 14.5123) -> (16.6136, 14.7368) centre (16.7259, 14.6246) ccw
  arc A4763 (14.6016, 26.2181) -> (14.895, 26.0966) centre (14.7483, 26.1574) ccw
  arc A4764 (16.2514, 24.4956) -> (16.2514, 24.8131) centre (16.2514, 24.6543) ccw
  arc A4765 (6.752, 31.4642) -> (6.752, 31.1467) centre (6.752, 31.3054) ccw
  line L1717 (6.8572, 19.7485) -> (7.62, 19.7485)
  arc A4766 (14.6245, 13.9129) -> (14.6245, 13.5954) centre (14.6245, 13.7542) ccw
  arc A4767 (13.5954, 14.6245) -> (13.9129, 14.6245) centre (13.7542, 14.6245) ccw
  arc A4768 (15.0514, 25.3101) -> (14.8269, 25.0856) centre (14.9391, 25.1979) ccw
  arc A4769 (15.3954, 26.8498) -> (15.1709, 27.0744) centre (15.2831, 26.9621) ccw
  arc A4770 (7.62, 23.5902) -> (7.62, 23.2727) centre (7.62, 23.4315) ccw
  line L1718 (9.4615, 22.3528) -> (8.3828, 23.4315)
  arc A4771 (6.8643, 31.1932) -> (6.6398, 31.4178) centre (6.7521, 31.3055) ccw
  arc A4772 (8.3828, 19.5897) -> (8.3828, 19.9073) centre (8.3828, 19.7485) ccw
  arc A4773 (7.7788, 21.59) -> (7.4613, 21.59) centre (7.6201, 21.59) ccw
  arc A4774 (15.3526, 24.9918) -> (15.2311, 24.6985) centre (15.2918, 24.8452) ccw
  arc A4775 (14.8269, 26.7304) -> (15.0514, 26.5059) centre (14.9391, 26.6182) ccw
  line L1719 (14.9392, 25.1978) -> (15.2918, 24.8452)
  arc A4776 (8.6955, 27.1209) -> (8.6955, 26.8034) centre (8.6955, 26.9622) ccw
  arc A4777 (9.6202, 21.59) -> (9.3027, 21.59) centre (9.4615, 21.59) ccw
  line L1720 (7.62, 23.4315) -> (7.62, 21.59)
  arc A4778 (15.0858, 26.5574) -> (14.7925, 26.6789) centre (14.9392, 26.6181) ccw
  line L1721 (15.8555, 13.7541) -> (16.7259, 14.6245)
  line L1722 (8.3325, 27.1145) -> (8.3361, 27.111)
  arc A4779 (7.7787, 23.4315) -> (7.4612, 23.4315) centre (7.62, 23.4315) ccw
  arc A4780 (5.7785, 21.7487) -> (5.7785, 21.4312) centre (5.7785, 21.59) ccw
  arc A4781 (14.895, 25.7194) -> (14.6016, 25.5979) centre (14.7483, 25.6587) ccw
  arc A4782 (5.8908, 20.9395) -> (5.6662, 20.715) centre (5.7785, 20.8272) ccw
  line L1723 (5.7785, 21.59) -> (7.62, 21.59)
  arc A4783 (14.5896, 25.6586) -> (14.907, 25.6586) centre (14.7483, 25.6586) ccw
  line L1724 (8.3361, 27.111) -> (8.6955, 26.9621)
  line L1725 (5.7785, 20.8272) -> (6.8572, 19.7485)
  arc A4784 (7.7787, 21.59) -> (7.4612, 21.59) centre (7.62, 21.59) ccw
  arc A4785 (7.4612, 21.59) -> (7.7787, 21.59) centre (7.62, 21.59) ccw
  arc A4786 (5.6197, 20.8272) -> (5.9373, 20.8272) centre (5.7785, 20.8272) ccw
  line L1726 (5.7785, 21.59) -> (5.7785, 20.8272)
  arc A4787 (6.752, 27.2733) -> (6.752, 26.9557) centre (6.752, 27.1145) ccw
  arc A4788 (8.488, 31.1467) -> (8.488, 31.4642) centre (8.488, 31.3054) ccw
  arc A4789 (8.6347, 26.8154) -> (8.7562, 27.1088) centre (8.6955, 26.9621) ccw
  line L1727 (16.2514, 24.6543) -> (16.5186, 24.765)
  arc A4790 (5.9373, 22.3528) -> (5.6197, 22.3528) centre (5.7785, 22.3528) ccw
  line L1728 (6.752, 31.3055) -> (5.5245, 30.078)
  line L1729 (28.1196, 23.4133) -> (28.2255, 23.3074)
  line L1730 (27.0211, 22.6949) -> (27.67, 22.9637)
  line L1731 (29.21, 25.4) -> (29.21, 22.9489)
  arc A4791 (16.5186, 24.9238) -> (16.5186, 24.6062) centre (16.5186, 24.765) ccw
  arc A4792 (8.2238, 26.9988) -> (8.4484, 27.2232) centre (8.3361, 27.111) ccw
  line L1732 (28.6299, 23.0596) -> (28.8561, 22.9861)
  line L1733 (9.7155, 30.078) -> (8.488, 31.3055)
  arc A4793 (29.21, 22.7902) -> (29.21, 23.1077) centre (29.21, 22.9489) ccw
  arc A4794 (15.6919, 24.5076) -> (15.8134, 24.801) centre (15.7527, 24.6543) ccw
  line L1734 (15.2831, 26.9621) -> (14.9392, 26.6182)
  arc A4795 (25.0514, 24.1698) -> (24.758, 24.0483) centre (24.9047, 24.109) ccw
  line L1735 (20.9425, 24.431) -> (21.3626, 24.257)
  arc A4796 (28.2319, 23.5255) -> (28.0073, 23.301) centre (28.1196, 23.4133) ccw
  line L1736 (6.752, 27.1145) -> (8.3325, 27.1145)
  line L1737 (5.5245, 28.342) -> (6.752, 27.1145)
  arc A4797 (28.1132, 23.1952) -> (28.3377, 23.4197) centre (28.2255, 23.3075) ccw
  arc A4798 (6.745, 19.6362) -> (6.9695, 19.8608) centre (6.8573, 19.7485) ccw
  arc A4799 (28.3246, 23.0392) -> (28.5112, 23.296) centre (28.4179, 23.1676) ccw
  line L1738 (20.6086, 24.765) -> (20.621, 24.7525)
  line L1739 (29.21, 22.9489) -> (29.21, 25.4)
  arc A4800 (16.5794, 24.6183) -> (16.4579, 24.9117) centre (16.5187, 24.765) ccw
  arc A4801 (16.1906, 24.801) -> (16.3121, 24.5076) centre (16.2514, 24.6543) ccw
  arc A4802 (24.9047, 24.0983) -> (24.9047, 24.4158) centre (24.9047, 24.2571) ccw
  line L1740 (28.4179, 23.1676) -> (28.6299, 23.0596)
  line L1741 (16.5186, 24.765) -> (20.6086, 24.765)
  arc A4803 (29.0662, 22.7921) -> (29.1159, 23.1057) centre (29.0911, 22.9489) ccw
  arc A4804 (6.6398, 27.0022) -> (6.8643, 27.2268) centre (6.7521, 27.1145) ccw
  arc A4805 (25.0268, 23.3995) -> (25.3201, 23.521) centre (25.1735, 23.4603) ccw
  arc A4806 (14.907, 26.1574) -> (14.5896, 26.1574) centre (14.7483, 26.1574) ccw
  line L1742 (20.621, 24.7525) -> (20.9425, 24.431)
  arc A4807 (5.6833, 30.078) -> (5.3658, 30.078) centre (5.5246, 30.078) ccw
  arc A4808 (5.9373, 21.59) -> (5.6197, 21.59) centre (5.7785, 21.59) ccw
  line L1743 (14.9392, 26.6182) -> (14.7483, 26.1574)
  arc A4809 (14.7925, 25.1371) -> (15.0858, 25.2586) centre (14.9392, 25.1979) ccw
  line L1744 (7.62, 21.59) -> (5.7785, 21.59)
  arc A4810 (7.62, 21.4313) -> (7.62, 21.7488) centre (7.62, 21.5901) ccw
  arc A4811 (5.6368, 28.4543) -> (5.4122, 28.2298) centre (5.5245, 28.3421) ccw
  arc A4812 (15.1796, 24.7329) -> (15.4041, 24.9574) centre (15.2919, 24.8452) ccw
  arc A4813 (15.2831, 26.8034) -> (15.2831, 27.1209) centre (15.2831, 26.9622) ccw
  line L1745 (5.5245, 30.078) -> (5.5245, 28.342)
  line L1746 (14.7483, 25.6586) -> (14.9392, 25.1978)
  arc A4814 (8.6002, 31.4178) -> (8.3757, 31.1932) centre (8.4879, 31.3055) ccw
  arc A4815 (5.3658, 28.342) -> (5.6833, 28.342) centre (5.5246, 28.342) ccw
  line L1747 (24.9047, 24.257) -> (24.9047, 24.1091)
  arc A4816 (21.3019, 24.1103) -> (21.4234, 24.4037) centre (21.3627, 24.257) ccw
  line L1748 (30.3004, 23.4133) -> (30.75, 22.9637)
  line L1749 (25.67, 22.9637) -> (26.3189, 22.6949)
  line L1750 (21.3626, 24.257) -> (24.9047, 24.257)
  arc A4817 (27.0211, 22.5361) -> (27.0211, 22.8537) centre (27.0211, 22.6949) ccw
  arc A4818 (28.8809, 23.1429) -> (28.8313, 22.8293) centre (28.8561, 22.9861) ccw
  arc A4819 (29.0513, 22.9489) -> (29.3688, 22.9489) centre (29.2101, 22.9489) ccw
  arc A4820 (24.746, 24.1091) -> (25.0635, 24.1091) centre (24.9048, 24.1091) ccw
  line L1751 (25.1735, 23.4602) -> (25.67, 22.9637)
  arc A4821 (21.0033, 24.5777) -> (20.8818, 24.2843) centre (20.9426, 24.431) ccw
  arc A4822 (25.0635, 24.257) -> (24.746, 24.257) centre (24.9048, 24.257) ccw
  arc A4823 (28.6789, 23.2106) -> (28.5808, 22.9086) centre (28.6298, 23.0596) ccw
  arc A4824 (25.2857, 23.5725) -> (25.0612, 23.348) centre (25.1735, 23.4603) ccw
  arc A4825 (28.5578, 22.9182) -> (28.7019, 23.2011) centre (28.6299, 23.0597) ccw
  line L1752 (35.29, 22.9637) -> (35.56, 23.2337)
  arc A4826 (29.21, 25.2412) -> (29.21, 25.5587) centre (29.21, 25.4) ccw
  arc A4827 (20.7333, 24.8648) -> (20.5088, 24.6403) centre (20.621, 24.7526) ccw
  arc A4828 (29.0512, 22.9489) -> (29.3687, 22.9489) centre (29.2099, 22.9489) ccw
  line L1753 (28.8561, 22.9861) -> (29.0911, 22.9489)
  line L1754 (28.2255, 23.3074) -> (28.4179, 23.1676)
  arc A4829 (35.1777, 23.0759) -> (35.4022, 22.8514) centre (35.29, 22.9637) ccw
  arc A4830 (25.7308, 23.1103) -> (25.6093, 22.817) centre (25.67, 22.9637) ccw
  line L1755 (37.1811, 22.6949) -> (37.83, 22.9637)
  arc A4831 (29.9088, 23.296) -> (30.0954, 23.0392) centre (30.0021, 23.1676) ccw
  arc A4832 (28.3188, 23.4359) -> (28.1321, 23.179) centre (28.2254, 23.3075) ccw
  arc A4833 (29.3687, 25.4) -> (29.0512, 25.4) centre (29.2099, 25.4) ccw
  arc A4834 (26.3189, 22.8537) -> (26.3189, 22.5361) centre (26.3189, 22.6949) ccw
  arc A4835 (20.8303, 24.3188) -> (21.0548, 24.5433) centre (20.9426, 24.431) ccw
  arc A4836 (25.5578, 22.8514) -> (25.7823, 23.0759) centre (25.67, 22.9637) ccw
  line L1756 (26.3189, 22.6949) -> (27.0211, 22.6949)
  arc A4837 (26.9604, 22.8416) -> (27.0819, 22.5482) centre (27.0211, 22.6949) ccw
  arc A4838 (21.3626, 24.4158) -> (21.3626, 24.0983) centre (21.3626, 24.2571) ccw
  line L1757 (27.67, 22.9637) -> (28.1196, 23.4133)
  arc A4839 (28.807, 22.8351) -> (28.9052, 23.1371) centre (28.8561, 22.9861) ccw
  line L1758 (33.29, 22.9637) -> (33.9389, 22.6949)
  arc A4840 (35.8908, 23.1103) -> (35.7693, 22.817) centre (35.83, 22.9637) ccw
  arc A4841 (29.0911, 23.1077) -> (29.0911, 22.7902) centre (29.0911, 22.9489) ccw
  arc A4842 (29.21, 25.5587) -> (29.21, 25.2412) centre (29.21, 25.4) ccw
  arc A4843 (27.5577, 23.0759) -> (27.7822, 22.8514) centre (27.67, 22.9637) ccw
  line L1759 (24.9047, 24.1091) -> (25.1735, 23.4602)
  arc A4844 (32.8107, 22.817) -> (32.6892, 23.1103) centre (32.7499, 22.9637) ccw
  arc A4845 (37.1811, 22.5361) -> (37.1811, 22.8537) centre (37.1811, 22.6949) ccw
  arc A4846 (29.5887, 22.8293) -> (29.5391, 23.1429) centre (29.5639, 22.9861) ccw
  arc A4847 (29.3041, 23.1057) -> (29.3538, 22.7921) centre (29.329, 22.9489) ccw
  arc A4848 (35.3507, 22.817) -> (35.2292, 23.1103) centre (35.29, 22.9637) ccw
  arc A4849 (28.49, 23.3091) -> (28.3458, 23.0262) centre (28.4179, 23.1677) ccw
  arc A4850 (30.6378, 22.8514) -> (30.8623, 23.0759) centre (30.7501, 22.9637) ccw
  line L1760 (32.75, 22.9637) -> (33.02, 23.2337)
  line L1761 (33.9389, 22.6949) -> (34.6411, 22.6949)
  arc A4851 (28.2319, 23.301) -> (28.0073, 23.5255) centre (28.1196, 23.4133) ccw
  arc A4852 (20.6086, 24.6062) -> (20.6086, 24.9238) centre (20.6086, 24.765) ccw
  arc A4853 (31.3381, 22.5482) -> (31.4596, 22.8416) centre (31.3989, 22.6949) ccw
  arc A4854 (26.2581, 22.5482) -> (26.3796, 22.8416) centre (26.3189, 22.6949) ccw
  arc A4855 (20.5088, 24.6403) -> (20.7333, 24.8648) centre (20.621, 24.7526) ccw
  line L1762 (30.75, 22.9637) -> (31.3989, 22.6949)
  arc A4856 (32.0404, 22.8416) -> (32.1619, 22.5482) centre (32.1012, 22.6949) ccw
  line L1763 (30.1945, 23.3074) -> (30.3004, 23.4133)
  arc A4857 (32.6377, 23.0759) -> (32.8622, 22.8514) centre (32.75, 22.9637) ccw
  line L1764 (29.5639, 22.9861) -> (29.7901, 23.0596)
  arc A4858 (34.6411, 22.5361) -> (34.6411, 22.8537) centre (34.6411, 22.6949) ccw
  arc A4859 (37.8907, 22.817) -> (37.7692, 23.1103) centre (37.83, 22.9637) ccw
  arc A4860 (20.7208, 24.8773) -> (20.4963, 24.6527) centre (20.6086, 24.765) ccw
  arc A4861 (27.7307, 22.817) -> (27.6092, 23.1103) centre (27.67, 22.9637) ccw
  line L1765 (29.0911, 22.9489) -> (29.21, 22.9489)
  arc A4862 (35.6723, 23.1214) -> (35.4477, 23.3459) centre (35.56, 23.2336) ccw
  line L1766 (33.9389, 28.1051) -> (33.29, 27.8363)
  arc A4863 (36.5396, 27.9584) -> (36.4181, 28.2518) centre (36.4789, 28.1051) ccw
  arc A4864 (38.4388, 23.348) -> (38.2143, 23.5725) centre (38.3266, 23.4603) ccw
  arc A4865 (33.9389, 22.8537) -> (33.9389, 22.5361) centre (33.9389, 22.6949) ccw
  arc A4866 (30.2879, 23.179) -> (30.1012, 23.4359) centre (30.1946, 23.3075) ccw
  arc A4867 (36.4181, 22.5482) -> (36.5396, 22.8416) centre (36.4789, 22.6949) ccw
  arc A4868 (31.3989, 22.8537) -> (31.3989, 22.5361) centre (31.3989, 22.6949) ccw
  arc A4869 (30.4126, 23.301) -> (30.1881, 23.5255) centre (30.3004, 23.4133) ccw
  arc A4870 (32.9077, 27.4541) -> (33.1323, 27.6786) centre (33.02, 27.5663) ccw
  arc A4871 (33.4023, 27.7241) -> (33.1778, 27.9486) centre (33.2901, 27.8364) ccw
  arc A4872 (35.2292, 27.6897) -> (35.3507, 27.983) centre (35.29, 27.8364) ccw
  line L1767 (34.6411, 22.6949) -> (35.29, 22.9637)
  arc A4873 (33.1323, 23.1214) -> (32.9077, 23.3459) centre (33.02, 23.2336) ccw
  arc A4874 (33.3508, 23.1103) -> (33.2293, 22.817) centre (33.2901, 22.9636) ccw
  arc A4875 (35.4477, 27.4541) -> (35.6723, 27.6786) centre (35.56, 27.5663) ccw
  arc A4876 (29.93, 27.4909) -> (30.0742, 27.7738) centre (30.0021, 27.6324) ccw
  line L1768 (38.5953, 24.1091) -> (38.5953, 26.6909)
  arc A4877 (37.1811, 27.9463) -> (37.1811, 28.2638) centre (37.1811, 28.1051) ccw
  line L1769 (33.29, 27.8363) -> (33.02, 27.5663)
  line L1770 (31.3989, 22.6949) -> (32.1011, 22.6949)
  line L1771 (35.56, 23.2337) -> (35.83, 22.9637)
  arc A4878 (33.9389, 28.2638) -> (33.9389, 27.9463) centre (33.9389, 28.1051) ccw
  arc A4879 (32.8622, 27.9486) -> (32.6377, 27.7241) centre (32.75, 27.8364) ccw
  arc A4880 (30.0954, 27.7608) -> (29.9088, 27.5039) centre (30.0021, 27.6324) ccw
  line L1772 (30.0021, 23.1676) -> (30.1945, 23.3074)
  arc A4881 (30.4126, 23.5255) -> (30.1881, 23.301) centre (30.3004, 23.4133) ccw
  arc A4882 (30.0742, 23.0262) -> (29.93, 23.3091) centre (30.0021, 23.1676) ccw
  arc A4883 (34.5804, 22.8416) -> (34.7019, 22.5482) centre (34.6412, 22.6949) ccw
  line L1773 (36.4789, 28.1051) -> (35.83, 27.8363)
  line L1774 (38.3265, 27.3398) -> (37.83, 27.8363)
  arc A4884 (37.1204, 22.8416) -> (37.2419, 22.5482) centre (37.1812, 22.6949) ccw
  arc A4885 (29.3289, 22.7902) -> (29.3289, 23.1077) centre (29.3289, 22.9489) ccw
  line L1775 (33.02, 23.2337) -> (33.29, 22.9637)
  arc A4886 (29.7181, 23.2011) -> (29.8622, 22.9182) centre (29.7902, 23.0597) ccw
  line L1776 (30.0021, 27.6324) -> (29.7901, 27.7404)
  arc A4887 (30.0823, 23.4197) -> (30.3068, 23.1952) centre (30.1946, 23.3075) ccw
  arc A4888 (33.1323, 23.3459) -> (32.9077, 23.1214) centre (33.02, 23.2336) ccw
  line L1777 (29.7901, 23.0596) -> (30.0021, 23.1676)
  arc A4889 (37.7177, 23.0759) -> (37.9422, 22.8514) centre (37.83, 22.9637) ccw
  arc A4890 (29.5148, 23.1371) -> (29.613, 22.8351) centre (29.5639, 22.9861) ccw
  arc A4891 (35.7178, 22.8514) -> (35.9423, 23.0759) centre (35.83, 22.9637) ccw
  line L1778 (29.7901, 27.7404) -> (29.5639, 27.8139)
  arc A4892 (30.8108, 23.1103) -> (30.6893, 22.817) centre (30.7501, 22.9637) ccw
  line L1779 (29.21, 22.9489) -> (29.3289, 22.9489)
  line L1780 (37.83, 22.9637) -> (38.3265, 23.4602)
  arc A4893 (36.4789, 22.8537) -> (36.4789, 22.5361) centre (36.4789, 22.6949) ccw
  arc A4894 (35.6723, 23.3459) -> (35.4477, 23.1214) centre (35.56, 23.2336) ccw
  arc A4895 (29.21, 23.1077) -> (29.21, 22.7902) centre (29.21, 22.9489) ccw
  arc A4896 (32.1011, 22.5361) -> (32.1011, 22.8537) centre (32.1011, 22.6949) ccw
  arc A4897 (33.8781, 22.5482) -> (33.9996, 22.8416) centre (33.9389, 22.6949) ccw
  line L1781 (35.83, 22.9637) -> (36.4789, 22.6949)
  arc A4898 (29.3688, 25.4) -> (29.0513, 25.4) centre (29.2101, 25.4) ccw
  line L1782 (29.3289, 22.9489) -> (29.5639, 22.9861)
  line L1783 (36.4789, 22.6949) -> (37.1811, 22.6949)
  arc A4899 (37.9422, 27.9486) -> (37.7177, 27.7241) centre (37.83, 27.8363) ccw
  arc A4900 (29.8392, 22.9086) -> (29.7411, 23.2106) centre (29.7902, 23.0596) ccw
  arc A4901 (38.1799, 23.521) -> (38.4732, 23.3995) centre (38.3266, 23.4603) ccw
  line L1784 (32.1011, 22.6949) -> (32.75, 22.9637)
  arc A4902 (33.1778, 22.8514) -> (33.4023, 23.0759) centre (33.2901, 22.9637) ccw
  line L1785 (35.56, 27.5663) -> (35.29, 27.8363)
  arc A4903 (29.8622, 27.8818) -> (29.7181, 27.5989) centre (29.7902, 27.7403) ccw
  line L1786 (28.4134, 29.337) -> (38.3274, 29.337)
  line L1787 (29.21, 25.4) -> (29.21, 27.8511)
  line L1788 (29.21, 27.8511) -> (29.0911, 27.8511)
  arc A4904 (28.3458, 27.7738) -> (28.49, 27.4909) centre (28.4179, 27.6324) ccw
  arc A4905 (30.3068, 27.6048) -> (30.0823, 27.3803) centre (30.1946, 27.4926) ccw
  arc A4906 (29.21, 28.0098) -> (29.21, 27.6923) centre (29.21, 27.8511) ccw
  line L1789 (32.75, 27.8363) -> (32.1011, 28.1051)
  arc A4907 (31.3989, 28.2638) -> (31.3989, 27.9463) centre (31.3989, 28.1051) ccw
  arc A4908 (28.1321, 27.621) -> (28.3188, 27.3641) centre (28.2254, 27.4926) ccw
  arc A4909 (33.9996, 27.9584) -> (33.8781, 28.2518) centre (33.9388, 28.1051) ccw
  arc A4910 (27.9253, 27.8056) -> (27.7007, 27.5811) centre (27.813, 27.6933) ccw
  arc A4911 (38.6352, 29.6233) -> (38.8597, 29.3988) centre (38.7475, 29.5111) ccw
  arc A4912 (29.0512, 25.4) -> (29.3687, 25.4) centre (29.2099, 25.4) ccw